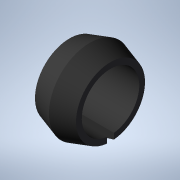
# Autodesk Inventor part: 61581400_3
Saved by Autodesk Inventor 2021 (Build 250183000, 183)
## iProperties
Created: 2026-05-06
Part Number: 61581400_3
Material: Generic
Catalog Web Link: www.3dfindit.com
Description: it_schrschei_st-Inner part, Shrink Disks ST, For very high torques
Vendor: MAEDLER
Document SubType Name: Modeling
Designer: psAdmin
Manufacturer: MAEDLER
Mass: 1.0889 g
Surface Area: 11.8678 cm^2
Volume: 1.0889 cm^3
Density: 1 g/cm^3
Appearance: PSOLRGB-176-176-176
Category: PARTsolutions
Company: MAEDLER
Title: 61581400
Author: Cadenas PARTsolutions
Comments: Inner part, Shrink Disks ST, For very high torques
PSOL_IDENT_0: {$CADENAS_DATA/23d-libs/maedler/antriebselemente/spannbuchsen_und_spannsaetze/schrumpfscheiben/schru
PSOL_IDENT_1: mpfscheibe_st/it_schrschei_st.prj},167 {VTYP=3D},{NB=61581400_3},{LINA=61581400},{NN=it_schrschei_st
PSOL_IDENT_2: },{DATE=03.01.2025 06:33:44},{GEOMDATE=03.01.2025 06:33:44},{VERSION=},{LINEID=20},{WBVAR=},{WBNUMER
PSOL_IDENT_3: IC=}  {NB=61581400_3},{LINA=61581400},{KT=DUMMY},{ARTNR=61581400},{WEBSHOP=Produktdetails / Katalogs
PSOL_IDENT_4: eite / Montageanleitung},{MATK=Stahl},{MAT=Hochwertiger Stahl 42CrMo4},{ID=14},{DW=10 / 11 / 12},{DM=
PSOL_IDENT_5: 40 / 50 / 65},{D=38},{L=15.0},{L2=18.5},{I=10},{E=2.50},{PSMAX=0.014},{SCHR= 4 x M5 x 12},{TA=3},{PW=
PSOL_IDENT_6: 154 / 191 / 243},{GEW=0.10},{TK=26.0},{SSA=4},{SSG=5},{SSL=12},{K=3.5},{SDW=6.9},{SW=8},{HDW=0.5},{D
PSOL_IDENT_7: G=5.3},{D1L=20.00},{D2L=16.80},{SL=1.70},{HD=35.6},{BA=6.650},{TN=it_schrschei_st_14},{CTN=84839089}
NB: 61581400_3
NN: it_schrschei_st
NT: Inner part, Shrink Disks ST, For very high torques
NBSYN: $ARTNR._3
LINA: 61581400
CATALOG: MÄDLER
ARTNR: 61581400
WEBSHOP: Produktdetails / Katalogseite / Montageanleitung
MATK: Stahl
MAT: Hochwertiger Stahl 42CrMo4
ID: 14
DW: 10 / 11 / 12
DM: 40 / 50 / 65
D: 38
L: 15
L2: 18.5
I: 10
E: 2.5
PSMAX: 0.014
SCHR: 4 x M5 x 12
TA: 3
PW: 154 / 191 / 243
GEW: 0.1
TK: 26
SSA: 4
SSG: 5
SSL: 12
K: 3.5
SDW: 6.9
SW: 8
HDW: 0.5
DG: 5.3
D1L: 20
D2L: 16.8
SL: 1.7
HD: 35.6
BA: 6.65
TN: it_schrschei_st_14
CTN: 84839089
SUPPLIER: MAEDLER
ARTICLENO: 61581400_3
BOMINFO: 61581400
CREATOR: CADENAS GmbH
Autodesk Inventor part; units mm, degrees
sketch "Sketch_5" plane through (0, 0, 0) normal (0, 0, 1) x (1, 0, 0)
  line L0 (500, 0) -> (-500, 0)
  line L1 (2.5, 8.4) -> (2.5, 7)
  line L2 (2.5, 7) -> (12.5, 7)
  line L3 (12.5, 7) -> (12.5, 8.4)
  line L4 (12.5, 8.4) -> (7.5, 10)
  line L5 (7.5, 10) -> (2.5, 8.4)
  constraints: 12 end point
revolve "Revolution1" add sketch "Sketch_5" angle 360 about axis through (500, 0, 0) along (1, 0, 0)
sketch "Sketch_6" plane through (7.5, 0, 0) normal (1, 0, 0) x (0, 0, -1)
  line L0 (-0.85, -10) -> (0.85, -10)
  line L1 (0.85, -10) -> (0.85, -6.5)
  line L2 (0.85, -6.5) -> (-0.85, -6.5)
  line L3 (-0.85, -6.5) -> (-0.85, -10)
  constraints: 8 end point
extrude "Extrusion1" cut sketch "Sketch_6" along normal mid plane 15
ref_plane "it_schrschei_st_XY" through (7.5, 0, 0) normal (1, 0, 0) x (0, 0, -1)
ref_plane "it_schrschei_st_YZ" through (7.5, 0, 0) normal (0, 0, -1) x (0, 1, 0)
ref_plane "it_schrschei_st_ZX" through (7.5, 0, 0) normal (0, 1, 0) x (1, 0, 0)
body "Solid1"
